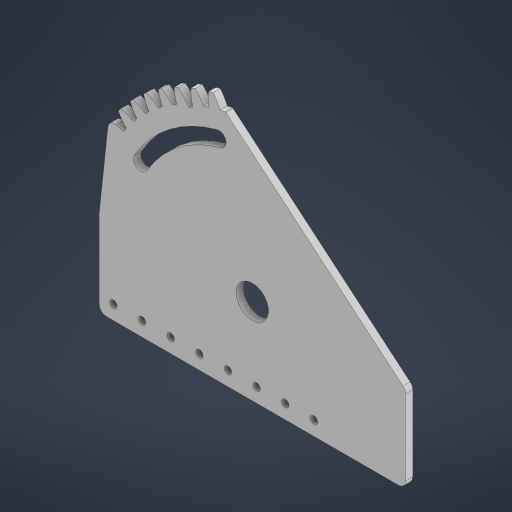
# Autodesk Inventor part: SHOT_0_001
Saved by Autodesk Inventor 2024.2 (Build 282272000, 272)
## iProperties
Created: 2024-08-07
Part Number: SHOT_0_001
Material: Generic
Document SubType Name: Modeling
Designer: Bryan
Density: 1 g/cm^3
Appearance: Default
Author: Bryan
Autodesk Inventor part; units mm, degrees
ref_plane "YZ Plane" through (0, 0, 0) normal (1, 0, 0) x (0, 1, 0)
ref_plane "XZ Plane" through (0, 0, 0) normal (0, 1, 0) x (-1, 0, 0)
ref_plane "XY Plane" through (0, 0, 0) normal (0, 0, 1) x (1, 0, 0)
sketch "Sketch2" plane through (0, 0, 0) normal (0, 0, 1) x (1, 0, 0)
  circle A0 centre (0, 0) radius 142.24 construction
  circle A1 centre (0, 0) radius 135.89
  circle A2 centre (0, 0) radius 147.32
  line L0 (0, 142.24) -> (0, 0) construction
  line L1 (0, 0) -> (-45.7151, 125.6011) construction
  line L2 (-45.7151, 125.6011) -> (0, 142.24) construction
  arc A3 (1.9921, 133.647) -> (-45.7151, 125.6011) centre (0, 0) ccw construction
  arc A4 (-45.7151, 125.6011) -> (-57.9663, 120.4384) centre (0, 0) ccw
  line L3 (-57.9663, 120.4384) -> (-2.146, 147.3044) construction
  spline S0 degree 2 poles (-2.146, 147.3044) (0.5723, 142.4261) (1.9921, 133.647) knots 0 0 0 1 1 1
  line L4 (0, 0) -> (3.8112, 135.8365) construction
  spline S1 degree 2 poles (10.4021, 146.9523) (7.4145, 142.2341) (5.5047, 133.5485) knots 0 0 0 1 1 1
  spline S2 degree 2 poles (-18.6254, 146.1379) (-15.3779, 141.5946) (-12.9842, 133.0297) knots 0 0 0 1 1 1
  spline S3 degree 2 poles (-6.1168, 147.193) (-8.5573, 142.1699) (-9.4826, 133.3251) knots 0 0 0 1 1 1
  spline S4 degree 2 poles (-34.8705, 143.1336) (-31.1348, 138.9825) (-27.7971, 130.7395) knots 0 0 0 1 1 1
  spline S5 degree 2 poles (-22.5587, 145.5826) (-24.4215, 140.3178) (-24.3506, 131.4251) knots 0 0 0 1 1 1
  spline S6 degree 2 poles (-50.6772, 138.3293) (-46.5001, 134.6226) (-42.2605, 126.8051) knots 0 0 0 1 1 1
  spline S7 degree 2 poles (-38.7169, 142.1414) (-39.9785, 136.7012) (-38.9125, 127.8723) knots 0 0 0 1 1 1
  spline S8 degree 2 poles (-65.8465, 131.7855) (-61.2807, 128.5698) (-56.1925, 121.2761) knots 0 0 0 1 1 1
  spline S9 degree 2 poles (-54.3883, 136.9127) (-55.0328, 131.3655) (-52.9849, 122.7114) knots 0 0 0 1 1 1
  spline S10 degree 2 poles (-80.1878, 123.5844) (-75.2906, 120.9001) (-69.4178, 114.222) knots 0 0 0 1 1 1
  spline S11 degree 2 poles (-69.3756, 129.9623) (-69.3951, 124.3778) (-66.3911, 116.0074) knots 0 0 0 1 1 1
  spline S12 degree 2 poles (-93.5206, 113.8292) (-88.3537, 111.71) (-81.7701, 105.7315) knots 0 0 0 1 1 1
  spline S13 degree 2 poles (-83.4906, 121.3775) (-82.8846, 115.8259) (-78.9624, 107.8445) knots 0 0 0 1 1 1
  spline S14 degree 2 poles (-105.6774, 102.6424) (-100.3057, 101.1151) (-93.0941, 95.9113) knots 0 0 0 1 1 1
  spline S15 degree 2 poles (-96.5556, 111.2664) (-95.3319, 105.8175) (-90.5406, 98.3255) knots 0 0 0 1 1 1
  spline S16 degree 2 poles (-116.5052, 90.1649) (-110.9963, 89.2486) (-103.2474, 84.885) knots 0 0 0 1 1 1
  spline S17 degree 2 poles (-108.4063, 99.7559) (-106.5802, 94.4784) (-100.9803, 87.5699) knots 0 0 0 1 1 1
  spline S18 degree 2 poles (-125.8679, 76.5535) (-120.2911, 76.2598) (-112.1023, 72.7912) knots 0 0 0 1 1 1
  spline S19 degree 2 poles (-118.8938, 86.991) (-116.4883, 81.9511) (-110.15, 75.713) knots 0 0 0 1 1 1
  spline S20 degree 2 poles (-133.6478, 61.9795) (-128.0731, 62.312) (-119.5475, 59.7821) knots 0 0 0 1 1 1
  spline S21 degree 2 poles (-127.8862, 73.1322) (-124.9315, 68.3933) (-117.9346, 62.9041) knots 0 0 0 1 1 1
  spline S22 degree 2 poles (-139.7469, 46.6259) (-134.2446, 47.5805) (-125.4893, 46.0211) knots 0 0 0 1 1 1
  spline S23 degree 2 poles (-135.2702, 58.3536) (-131.8035, 53.9753) (-124.2361, 49.3041) knots 0 0 0 1 1 1
  spline S24 degree 2 poles (-144.0887, 30.6861) (-138.7278, 32.2507) (-129.8529, 31.6814) knots 0 0 0 1 1 1
  spline S25 degree 2 poles (-140.9532, 42.8412) (-137.0181, 38.8786) (-128.9752, 35.084) knots 0 0 0 1 1 1
  spline S26 degree 2 poles (-146.6184, 14.3603) (-141.4664, 16.5154) (-132.5836, 16.9433) knots 0 0 0 1 1 1
  spline S27 degree 2 poles (-144.8636, 26.7901) (-140.5096, 23.293) (-132.0924, 20.4228) knots 0 0 0 1 1 1
  spline S28 degree 2 poles (-147.3044, -2.146) (-142.4261, 0.5723) (-133.647, 1.9921) knots 0 0 0 1 1 1
  spline S29 degree 2 poles (-146.9523, 10.4021) (-142.2341, 7.4145) (-133.5485, 5.5047) knots 0 0 0 1 1 1
  spline S30 degree 2 poles (-146.1379, -18.6254) (-141.5946, -15.3779) (-133.0297, -12.9842) knots 0 0 0 1 1 1
  spline S31 degree 2 poles (-147.193, -6.1168) (-142.1699, -8.5573) (-133.3251, -9.4826) knots 0 0 0 1 1 1
  spline S32 degree 2 poles (-143.1336, -34.8705) (-138.9825, -31.1348) (-130.7395, -27.7971) knots 0 0 0 1 1 1
  spline S33 degree 2 poles (-145.5826, -22.5587) (-140.3178, -24.4215) (-131.4251, -24.3506) knots 0 0 0 1 1 1
  spline S34 degree 2 poles (-138.3293, -50.6772) (-134.6226, -46.5001) (-126.8051, -42.2605) knots 0 0 0 1 1 1
  spline S35 degree 2 poles (-142.1414, -38.7169) (-136.7012, -39.9785) (-127.8723, -38.9125) knots 0 0 0 1 1 1
  spline S36 degree 2 poles (-131.7855, -65.8465) (-128.5698, -61.2807) (-121.2761, -56.1925) knots 0 0 0 1 1 1
  spline S37 degree 2 poles (-136.9127, -54.3883) (-131.3655, -55.0328) (-122.7114, -52.9849) knots 0 0 0 1 1 1
  spline S38 degree 2 poles (-123.5844, -80.1878) (-120.9001, -75.2906) (-114.222, -69.4178) knots 0 0 0 1 1 1
  spline S39 degree 2 poles (-129.9623, -69.3756) (-124.3778, -69.3951) (-116.0074, -66.3911) knots 0 0 0 1 1 1
  spline S40 degree 2 poles (-113.8292, -93.5206) (-111.71, -88.3537) (-105.7315, -81.7701) knots 0 0 0 1 1 1
  spline S41 degree 2 poles (-121.3775, -83.4906) (-115.8259, -82.8846) (-107.8445, -78.9624) knots 0 0 0 1 1 1
  spline S42 degree 2 poles (-102.6424, -105.6774) (-101.1151, -100.3057) (-95.9113, -93.0941) knots 0 0 0 1 1 1
  spline S43 degree 2 poles (-111.2664, -96.5556) (-105.8175, -95.3319) (-98.3255, -90.5406) knots 0 0 0 1 1 1
  spline S44 degree 2 poles (-90.1649, -116.5052) (-89.2486, -110.9963) (-84.885, -103.2474) knots 0 0 0 1 1 1
  spline S45 degree 2 poles (-99.7559, -108.4063) (-94.4784, -106.5802) (-87.5699, -100.9803) knots 0 0 0 1 1 1
  spline S46 degree 2 poles (-76.5535, -125.8679) (-76.2598, -120.2911) (-72.7912, -112.1023) knots 0 0 0 1 1 1
  spline S47 degree 2 poles (-86.991, -118.8938) (-81.9511, -116.4883) (-75.713, -110.15) knots 0 0 0 1 1 1
  spline S48 degree 2 poles (-61.9795, -133.6478) (-62.312, -128.0731) (-59.7821, -119.5475) knots 0 0 0 1 1 1
  spline S49 degree 2 poles (-73.1322, -127.8862) (-68.3933, -124.9315) (-62.9041, -117.9346) knots 0 0 0 1 1 1
  spline S50 degree 2 poles (-46.6259, -139.7469) (-47.5805, -134.2446) (-46.0211, -125.4893) knots 0 0 0 1 1 1
  spline S51 degree 2 poles (-58.3536, -135.2702) (-53.9753, -131.8035) (-49.3041, -124.2361) knots 0 0 0 1 1 1
  spline S52 degree 2 poles (-30.6861, -144.0887) (-32.2507, -138.7278) (-31.6814, -129.8529) knots 0 0 0 1 1 1
  spline S53 degree 2 poles (-42.8412, -140.9532) (-38.8786, -137.0181) (-35.084, -128.9752) knots 0 0 0 1 1 1
  spline S54 degree 2 poles (-14.3603, -146.6184) (-16.5154, -141.4664) (-16.9433, -132.5836) knots 0 0 0 1 1 1
  spline S55 degree 2 poles (-26.7901, -144.8636) (-23.293, -140.5096) (-20.4228, -132.0924) knots 0 0 0 1 1 1
  spline S56 degree 2 poles (2.146, -147.3044) (-0.5723, -142.4261) (-1.9921, -133.647) knots 0 0 0 1 1 1
  spline S57 degree 2 poles (-10.4021, -146.9523) (-7.4145, -142.2341) (-5.5047, -133.5485) knots 0 0 0 1 1 1
  spline S58 degree 2 poles (18.6254, -146.1379) (15.3779, -141.5946) (12.9842, -133.0297) knots 0 0 0 1 1 1
  spline S59 degree 2 poles (6.1168, -147.193) (8.5573, -142.1699) (9.4826, -133.3251) knots 0 0 0 1 1 1
  spline S60 degree 2 poles (34.8705, -143.1336) (31.1348, -138.9825) (27.7971, -130.7395) knots 0 0 0 1 1 1
  spline S61 degree 2 poles (22.5587, -145.5826) (24.4215, -140.3178) (24.3506, -131.4251) knots 0 0 0 1 1 1
  spline S62 degree 2 poles (50.6772, -138.3293) (46.5001, -134.6226) (42.2605, -126.8051) knots 0 0 0 1 1 1
  spline S63 degree 2 poles (38.7169, -142.1414) (39.9785, -136.7012) (38.9125, -127.8723) knots 0 0 0 1 1 1
  spline S64 degree 2 poles (65.8465, -131.7855) (61.2807, -128.5698) (56.1925, -121.2761) knots 0 0 0 1 1 1
  spline S65 degree 2 poles (54.3883, -136.9127) (55.0328, -131.3655) (52.9849, -122.7114) knots 0 0 0 1 1 1
  spline S66 degree 2 poles (80.1878, -123.5844) (75.2906, -120.9001) (69.4178, -114.222) knots 0 0 0 1 1 1
  spline S67 degree 2 poles (69.3756, -129.9623) (69.3951, -124.3778) (66.3911, -116.0074) knots 0 0 0 1 1 1
  spline S68 degree 2 poles (93.5206, -113.8292) (88.3537, -111.71) (81.7701, -105.7315) knots 0 0 0 1 1 1
  spline S69 degree 2 poles (83.4906, -121.3775) (82.8846, -115.8259) (78.9624, -107.8445) knots 0 0 0 1 1 1
  spline S70 degree 2 poles (105.6774, -102.6424) (100.3057, -101.1151) (93.0941, -95.9113) knots 0 0 0 1 1 1
  spline S71 degree 2 poles (96.5556, -111.2664) (95.3319, -105.8175) (90.5406, -98.3255) knots 0 0 0 1 1 1
  spline S72 degree 2 poles (116.5052, -90.1649) (110.9963, -89.2486) (103.2474, -84.885) knots 0 0 0 1 1 1
  spline S73 degree 2 poles (108.4063, -99.7559) (106.5802, -94.4784) (100.9803, -87.5699) knots 0 0 0 1 1 1
  spline S74 degree 2 poles (125.8679, -76.5535) (120.2911, -76.2598) (112.1023, -72.7912) knots 0 0 0 1 1 1
  spline S75 degree 2 poles (118.8938, -86.991) (116.4883, -81.9511) (110.15, -75.713) knots 0 0 0 1 1 1
  spline S76 degree 2 poles (133.6478, -61.9795) (128.0731, -62.312) (119.5475, -59.7821) knots 0 0 0 1 1 1
  spline S77 degree 2 poles (127.8862, -73.1322) (124.9315, -68.3933) (117.9346, -62.9041) knots 0 0 0 1 1 1
  spline S78 degree 2 poles (139.7469, -46.6259) (134.2446, -47.5805) (125.4893, -46.0211) knots 0 0 0 1 1 1
  spline S79 degree 2 poles (135.2702, -58.3536) (131.8035, -53.9753) (124.2361, -49.3041) knots 0 0 0 1 1 1
  spline S80 degree 2 poles (144.0887, -30.6861) (138.7278, -32.2507) (129.8529, -31.6814) knots 0 0 0 1 1 1
  spline S81 degree 2 poles (140.9532, -42.8412) (137.0181, -38.8786) (128.9752, -35.084) knots 0 0 0 1 1 1
  spline S82 degree 2 poles (146.6184, -14.3603) (141.4664, -16.5154) (132.5836, -16.9433) knots 0 0 0 1 1 1
  spline S83 degree 2 poles (144.8636, -26.7901) (140.5096, -23.293) (132.0924, -20.4228) knots 0 0 0 1 1 1
  spline S84 degree 2 poles (147.3044, 2.146) (142.4261, -0.5723) (133.647, -1.9921) knots 0 0 0 1 1 1
  spline S85 degree 2 poles (146.9523, -10.4021) (142.2341, -7.4145) (133.5485, -5.5047) knots 0 0 0 1 1 1
  spline S86 degree 2 poles (146.1379, 18.6254) (141.5946, 15.3779) (133.0297, 12.9842) knots 0 0 0 1 1 1
  spline S87 degree 2 poles (147.193, 6.1168) (142.1699, 8.5573) (133.3251, 9.4826) knots 0 0 0 1 1 1
  spline S88 degree 2 poles (143.1336, 34.8705) (138.9825, 31.1348) (130.7395, 27.7971) knots 0 0 0 1 1 1
  spline S89 degree 2 poles (145.5826, 22.5587) (140.3178, 24.4215) (131.4251, 24.3506) knots 0 0 0 1 1 1
  spline S90 degree 2 poles (138.3293, 50.6772) (134.6226, 46.5001) (126.8051, 42.2605) knots 0 0 0 1 1 1
  spline S91 degree 2 poles (142.1414, 38.7169) (136.7012, 39.9785) (127.8723, 38.9125) knots 0 0 0 1 1 1
  spline S92 degree 2 poles (131.7855, 65.8465) (128.5698, 61.2807) (121.2761, 56.1925) knots 0 0 0 1 1 1
  spline S93 degree 2 poles (136.9127, 54.3883) (131.3655, 55.0328) (122.7114, 52.9849) knots 0 0 0 1 1 1
  spline S94 degree 2 poles (123.5844, 80.1878) (120.9001, 75.2906) (114.222, 69.4178) knots 0 0 0 1 1 1
  spline S95 degree 2 poles (129.9623, 69.3756) (124.3778, 69.3951) (116.0074, 66.3911) knots 0 0 0 1 1 1
  spline S96 degree 2 poles (113.8292, 93.5206) (111.71, 88.3537) (105.7315, 81.7701) knots 0 0 0 1 1 1
  spline S97 degree 2 poles (121.3775, 83.4906) (115.8259, 82.8846) (107.8445, 78.9624) knots 0 0 0 1 1 1
  spline S98 degree 2 poles (102.6424, 105.6774) (101.1151, 100.3057) (95.9113, 93.0941) knots 0 0 0 1 1 1
  spline S99 degree 2 poles (111.2664, 96.5556) (105.8175, 95.3319) (98.3255, 90.5406) knots 0 0 0 1 1 1
  spline S100 degree 2 poles (90.1649, 116.5052) (89.2486, 110.9963) (84.885, 103.2474) knots 0 0 0 1 1 1
  spline S101 degree 2 poles (99.7559, 108.4063) (94.4784, 106.5802) (87.5699, 100.9803) knots 0 0 0 1 1 1
  spline S102 degree 2 poles (76.5535, 125.8679) (76.2598, 120.2911) (72.7912, 112.1023) knots 0 0 0 1 1 1
  spline S103 degree 2 poles (86.991, 118.8938) (81.9511, 116.4883) (75.713, 110.15) knots 0 0 0 1 1 1
  spline S104 degree 2 poles (61.9795, 133.6478) (62.312, 128.0731) (59.7821, 119.5475) knots 0 0 0 1 1 1
  spline S105 degree 2 poles (73.1322, 127.8862) (68.3933, 124.9315) (62.9041, 117.9346) knots 0 0 0 1 1 1
  spline S106 degree 2 poles (46.6259, 139.7469) (47.5805, 134.2446) (46.0211, 125.4893) knots 0 0 0 1 1 1
  spline S107 degree 2 poles (58.3536, 135.2702) (53.9753, 131.8035) (49.3041, 124.2361) knots 0 0 0 1 1 1
  spline S108 degree 2 poles (30.6861, 144.0887) (32.2507, 138.7278) (31.6814, 129.8529) knots 0 0 0 1 1 1
  spline S109 degree 2 poles (42.8412, 140.9532) (38.8786, 137.0181) (35.084, 128.9752) knots 0 0 0 1 1 1
  spline S110 degree 2 poles (14.3603, 146.6184) (16.5154, 141.4664) (16.9433, 132.5836) knots 0 0 0 1 1 1
  spline S111 degree 2 poles (26.7901, 144.8636) (23.293, 140.5096) (20.4228, 132.0924) knots 0 0 0 1 1 1
  circle A5 centre (0, 0) radius 6.35
  point P0 (7.9755, 142.0162)
  point P1 (-15.9258, 141.3456)
  point P2 (-7.9755, 142.0162)
  point P3 (-31.6514, 138.6737)
  point P4 (-23.8261, 140.2303)
  point P5 (-46.9789, 134.258)
  point P6 (-39.3771, 136.6809)
  point P7 (-61.7156, 128.1538)
  point P8 (-54.4329, 131.4126)
  point P9 (-75.6762, 120.4381)
  point P10 (-68.8042, 124.4918)
  point P11 (-88.6852, 111.2077)
  point P12 (-82.3102, 116.0054)
  point P13 (-100.5789, 100.5789)
  point P14 (-94.7811, 106.0601)
  point P15 (-111.2077, 88.6852)
  point P16 (-106.0601, 94.7811)
  point P17 (-120.4381, 75.6762)
  point P18 (-116.0054, 82.3102)
  point P19 (-128.1538, 61.7156)
  point P20 (-124.4918, 68.8042)
  point P21 (-134.258, 46.9789)
  point P22 (-131.4126, 54.4329)
  point P23 (-138.6737, 31.6514)
  point P24 (-136.6809, 39.3771)
  point P25 (-141.3456, 15.9258)
  point P26 (-140.2303, 23.8261)
  point P27 (-142.24, 0)
  point P28 (-142.0162, 7.9755)
  point P29 (-141.3456, -15.9258)
  point P30 (-142.0162, -7.9755)
  point P31 (-138.6737, -31.6514)
  point P32 (-140.2303, -23.8261)
  point P33 (-134.258, -46.9789)
  point P34 (-136.6809, -39.3771)
  point P35 (-128.1538, -61.7156)
  point P36 (-131.4126, -54.4329)
  point P37 (-120.4381, -75.6762)
  point P38 (-124.4918, -68.8042)
  point P39 (-111.2077, -88.6852)
  point P40 (-116.0054, -82.3102)
  point P41 (-100.5789, -100.5789)
  point P42 (-106.0601, -94.7811)
  point P43 (-88.6852, -111.2077)
  point P44 (-94.7811, -106.0601)
  point P45 (-75.6762, -120.4381)
  point P46 (-82.3102, -116.0054)
  point P47 (-61.7156, -128.1538)
  point P48 (-68.8042, -124.4918)
  point P49 (-46.9789, -134.258)
  point P50 (-54.4329, -131.4126)
  point P51 (-31.6514, -138.6737)
  point P52 (-39.3771, -136.6809)
  point P53 (-15.9258, -141.3456)
  point P54 (-23.8261, -140.2303)
  point P55 (0, -142.24)
  point P56 (-7.9755, -142.0162)
  point P57 (15.9258, -141.3456)
  point P58 (7.9755, -142.0162)
  point P59 (31.6514, -138.6737)
  point P60 (23.8261, -140.2303)
  point P61 (46.9789, -134.258)
  point P62 (39.3771, -136.6809)
  point P63 (61.7156, -128.1538)
  point P64 (54.4329, -131.4126)
  point P65 (75.6762, -120.4381)
  point P66 (68.8042, -124.4918)
  point P67 (88.6852, -111.2077)
  point P68 (82.3102, -116.0054)
  point P69 (100.5789, -100.5789)
  point P70 (94.7811, -106.0601)
  point P71 (111.2077, -88.6852)
  point P72 (106.0601, -94.7811)
  point P73 (120.4381, -75.6762)
  point P74 (116.0054, -82.3102)
  point P75 (128.1538, -61.7156)
  point P76 (124.4918, -68.8042)
  point P77 (134.258, -46.9789)
  point P78 (131.4126, -54.4329)
  point P79 (138.6737, -31.6514)
  point P80 (136.6809, -39.3771)
  point P81 (141.3456, -15.9258)
  point P82 (140.2303, -23.8261)
  point P83 (142.24, 0)
  point P84 (142.0162, -7.9755)
  point P85 (141.3456, 15.9258)
  point P86 (142.0162, 7.9755)
  point P87 (138.6737, 31.6514)
  point P88 (140.2303, 23.8261)
  point P89 (134.258, 46.9789)
  point P90 (136.6809, 39.3771)
  point P91 (128.1538, 61.7156)
  point P92 (131.4126, 54.4329)
  point P93 (120.4381, 75.6762)
  point P94 (124.4918, 68.8042)
  point P95 (111.2077, 88.6852)
  point P96 (116.0054, 82.3102)
  point P97 (100.5789, 100.5789)
  point P98 (106.0601, 94.7811)
  point P99 (88.6852, 111.2077)
  point P100 (94.7811, 106.0601)
  point P101 (75.6762, 120.4381)
  point P102 (82.3102, 116.0054)
  point P103 (61.7156, 128.1538)
  point P104 (68.8042, 124.4918)
  point P105 (46.9789, 134.258)
  point P106 (54.4329, 131.4126)
  point P107 (31.6514, 138.6737)
  point P108 (39.3771, 136.6809)
  point P109 (15.9258, 141.3456)
  point P110 (23.8261, 140.2303)
  point P111 (-52.9849, 122.7114)
  point P112 (-56.1925, 121.2761)
  point P113 (-65.8465, 131.7855)
  point P114 (-67.1264, 118.153)
  point P115 (-70.94, 115.9034)
  point P116 (-80.1878, 123.5844)
  point P117 (-79.9333, 109.8943)
  point P118 (-83.471, 107.2319)
  point P119 (-93.5206, 113.8292)
  point P120 (-96.5556, 111.2664)
  point P121 (-91.7349, 100.2537)
  point P122 (-94.9523, 97.2119)
  point P123 (-108.4063, 99.7559)
  point P124 (-102.383, 89.3522)
  point P125 (-105.2396, 85.9693)
  point P126 (-116.5052, 90.1649)
  point P127 (-118.8938, 86.991)
  point P128 (-111.7435, 77.3272)
  point P129 (-114.2034, 73.6457)
  point P130 (-125.8679, 76.5535)
  point P131 (-127.8862, 73.1322)
  point P132 (-119.6987, 64.3296)
  point P133 (-121.731, 60.3959)
  point P134 (-133.6478, 61.9795)
  point P135 (-135.2702, 58.3536)
  point P136 (-126.1487, 50.5231)
  point P137 (-127.7277, 46.3866)
  point P138 (-139.7469, 46.6259)
  point P139 (-140.9532, 42.8412)
  point P140 (-131.0123, 36.0813)
  point P141 (-132.1183, 31.794)
  point P142 (-144.0887, 30.6861)
  point P143 (-144.8636, 26.7901)
  point P144 (-134.2284, 21.1857)
  point P145 (-134.8473, 16.8015)
  point P146 (-146.6184, 14.3603)
  point P147 (-135.7564, 6.0237)
  point P148 (123.1174, 57.5169)
  point P149 (131.7855, 65.8465)
  point P150 (129.9623, 69.3756)
  point P151 (118.153, 67.1264)
  point P152 (115.9034, 70.94)
  point P153 (123.5844, 80.1878)
  point P154 (121.3775, 83.4906)
  point P155 (109.8943, 79.9333)
  point P156 (107.2319, 83.471)
  point P157 (113.8292, 93.5206)
  point P158 (111.2664, 96.5556)
  point P159 (100.2537, 91.7349)
  point P160 (97.2119, 94.9523)
  point P161 (102.6424, 105.6774)
  point P162 (99.7559, 108.4063)
  point P163 (89.3522, 102.383)
  point P164 (85.9693, 105.2396)
  point P165 (90.1649, 116.5052)
  point P166 (86.991, 118.8938)
  point P167 (77.3272, 111.7435)
  point P168 (73.6457, 114.2034)
  point P169 (76.5535, 125.8679)
  point P170 (73.1322, 127.8862)
  point P171 (64.3296, 119.6987)
  point P172 (60.3959, 121.731)
  point P173 (61.9795, 133.6478)
  point P174 (58.3536, 135.2702)
  point P175 (50.5231, 126.1487)
  point P176 (46.3866, 127.7277)
  point P177 (46.6259, 139.7469)
  point P178 (42.8412, 140.9532)
  point P179 (36.0813, 131.0123)
  point P180 (31.794, 132.1183)
  point P181 (30.6861, 144.0887)
  point P182 (26.7901, 144.8636)
  point P183 (21.1857, 134.2284)
  point P184 (16.8015, 134.8473)
  point P185 (14.3603, 146.6184)
  point P186 (6.0237, 135.7564)
  point P187 (1.5977, 135.8806)
  point P188 (-6.1168, 147.193)
  point P189 (-9.2141, 135.5773)
  point P190 (-13.6261, 135.2051)
  point P191 (-18.6254, 146.1379)
  point P192 (-24.336, 133.6931)
  point P193 (-28.6786, 132.8293)
  point P194 (-34.8705, 143.1336)
  point P195 (-39.1519, 130.1277)
  point P196 (-43.3704, 128.7831)
  point P197 (-50.6772, 138.3293)
  point P198 (-54.3883, 136.9127)
  dimension "d0" = 284.48
  dimension "d1" = 271.78
  dimension "d2" = 294.64
  dimension "d3" = 20
  dimension "d4" = 48.6489
  dimension "d5" = 48.6489
  dimension "d6" = 61.949
  dimension "d7" = 13.3001
  dimension "d8" = 1.607
  dimension "d11" = 360
  dimension "d13" = 12.7
  constraints: 10 end point, 4 coincident, 4 point on circle, 3 centre point, 3 symmetric about line, 1 perpendicular, 1 tangent, 1 vertical, 1 vertical alignment, 795 other
  measures "d3" angle of L0 L1
  measures "d4" distance of L1.end L0.start
  measures "d6" distance of L3.start L3.end
  measures "d8" angle of L4 L0
  measures "d13" diameter of A5
extrude "Extrusion1" add sketch "Sketch2" along normal blind 6.35 contours A1 S8 A4 S9 | A1 S95 A2 S92 | A1 S97 A2 S94 | A1 S99 A2 S96 | A1 S101 A2 S98 | A1 S103 A2 S100 | A1 S105 A2 S102 | A1 S107 A2 S104 | A1 S109 A2 S106 | A1 S111 A2 S108 | A1 S1 A2 S110 | A1 S3 A2 S0 | A1 S5 A2 S2 | A1 S7 A2 S4 | A1 S9 A2 S6 | A1 S11 A2 S8 | A1 S13 A2 S10 | A1 S15 A2 S12 | A1 S17 A2 S14 | A1 S19 A2 S16 | A1 S21 A2 S18 | A1 S23 A2 S20 | A1 S25 A2 S22 | A1 S27 A2 S24 | A1 S29 A2 S26 picked at (-28.6478, 87.0122)
sketch "Sketch3" plane through (0, 0, 6.35) normal (0, 0, 1) x (1, 0, 0)
  circle A0 centre (0, 0) radius 6.35 projected
  line L0 (0, 0) -> (-127.5829, 73.66)
  line L1 (0, 0) -> (-25.5818, 145.0819)
  line L2 (0, 0) -> (-135.89, 0) construction
  arc A1 (-135.7564, 6.0237) -> (123.1174, 57.5169) centre (0, 0) ccw projected
  line L3 (-135.89, 0) -> (-135.89, -76.2)
  line L4 (135.89, 0) -> (135.89, -76.2)
  line L5 (-135.89, -50.8) -> (135.89, -50.8)
  line L6 (-135.89, -76.2) -> (135.89, -76.2)
  arc A2 (-52.9849, 122.7114) -> (-56.1925, 121.2761) centre (0, 0) ccw projected
  arc A3 (-65.8465, 131.7855) -> (-69.3756, 129.9623) centre (0, 0) ccw projected
  arc A4 (-67.1264, 118.153) -> (-70.94, 115.9034) centre (0, 0) ccw projected
  arc A5 (-80.1878, 123.5844) -> (-83.4906, 121.3775) centre (0, 0) ccw projected
  arc A6 (-79.9333, 109.8943) -> (-83.471, 107.2319) centre (0, 0) ccw projected
  arc A7 (-93.5206, 113.8292) -> (-96.5556, 111.2664) centre (0, 0) ccw projected
  arc A8 (-91.7349, 100.2537) -> (-94.9523, 97.2119) centre (0, 0) ccw projected
  arc A9 (-105.6774, 102.6424) -> (-108.4063, 99.7559) centre (0, 0) ccw projected
  arc A10 (-102.383, 89.3522) -> (-105.2396, 85.9693) centre (0, 0) ccw projected
  arc A11 (-116.5052, 90.1649) -> (-118.8938, 86.991) centre (0, 0) ccw projected
  arc A12 (-111.7435, 77.3272) -> (-114.2034, 73.6457) centre (0, 0) ccw projected
  arc A13 (-125.8679, 76.5535) -> (-127.8862, 73.1322) centre (0, 0) ccw projected
  spline S0 degree 2 poles (-127.8862, 73.1322) (-125.3186, 69.0142) (-119.6987, 64.3296) knots 0 0 0 1 1 1 projected
  arc A14 (-119.6987, 64.3296) -> (-121.731, 60.3959) centre (0, 0) ccw projected
  spline S1 degree 2 poles (-121.731, 60.3959) (-128.8035, 62.2684) (-133.6478, 61.9795) knots 0 0 0 1 1 1 projected
  arc A15 (-133.6478, 61.9795) -> (-135.2702, 58.3536) centre (0, 0) ccw projected
  spline S2 degree 2 poles (-135.2702, 58.3536) (-132.2578, 54.549) (-126.1487, 50.5231) knots 0 0 0 1 1 1 projected
  arc A16 (-126.1487, 50.5231) -> (-127.7277, 46.3866) centre (0, 0) ccw projected
  spline S3 degree 2 poles (-127.7277, 46.3866) (-134.9655, 47.4555) (-139.7469, 46.6259) knots 0 0 0 1 1 1 projected
  arc A17 (-139.7469, 46.6259) -> (-140.9532, 42.8412) centre (0, 0) ccw projected
  spline S4 degree 2 poles (-140.9532, 42.8412) (-137.5337, 39.3978) (-131.0123, 36.0813) knots 0 0 0 1 1 1 projected
  arc A18 (-131.0123, 36.0813) -> (-132.1183, 31.794) centre (0, 0) ccw projected
  spline S5 degree 2 poles (-132.1183, 31.794) (-139.4302, 32.0457) (-144.0887, 30.6861) knots 0 0 0 1 1 1 projected
  arc A19 (-144.0887, 30.6861) -> (-144.8636, 26.7901) centre (0, 0) ccw projected
  spline S6 degree 2 poles (-144.8636, 26.7901) (-141.0801, 23.7512) (-134.2284, 21.1857) knots 0 0 0 1 1 1 projected
  arc A20 (-134.2284, 21.1857) -> (-134.8473, 16.8015) centre (0, 0) ccw projected
  spline S7 degree 2 poles (-134.8473, 16.8015) (-142.1415, 16.233) (-146.6184, 14.3603) knots 0 0 0 1 1 1 projected
  arc A21 (-146.6184, 14.3603) -> (-146.9523, 10.4021) centre (0, 0) ccw projected
  spline S8 degree 2 poles (-146.9523, 10.4021) (-142.8523, 7.8059) (-135.7564, 6.0237) knots 0 0 0 1 1 1 projected
  arc A22 (-135.7564, 6.0237) -> (123.1174, 57.5169) centre (0, 0) ccw projected
  spline S9 degree 2 poles (123.1174, 57.5169) (128.9911, 61.8789) (131.7855, 65.8465) knots 0 0 0 1 1 1 projected
  arc A23 (131.7855, 65.8465) -> (129.9623, 69.3756) centre (0, 0) ccw projected
  spline S10 degree 2 poles (129.9623, 69.3756) (125.1095, 69.3925) (118.153, 67.1264) knots 0 0 0 1 1 1 projected
  arc A24 (118.153, 67.1264) -> (115.9034, 70.94) centre (0, 0) ccw projected
  spline S11 degree 2 poles (115.9034, 70.94) (121.2518, 75.9323) (123.5844, 80.1878) knots 0 0 0 1 1 1 projected
  arc A25 (123.5844, 80.1878) -> (121.3775, 83.4906) centre (0, 0) ccw projected
  spline S12 degree 2 poles (121.3775, 83.4906) (116.5533, 82.964) (109.8943, 79.9333) knots 0 0 0 1 1 1 projected
  arc A26 (109.8943, 79.9333) -> (107.2319, 83.471) centre (0, 0) ccw projected
  spline S13 degree 2 poles (107.2319, 83.471) (111.9877, 89.0307) (113.8292, 93.5206) knots 0 0 0 1 1 1 projected
  arc A27 (113.8292, 93.5206) -> (111.2664, 96.5556) centre (0, 0) ccw projected
  spline S14 degree 2 poles (111.2664, 96.5556) (106.5314, 95.4922) (100.2537, 91.7349) knots 0 0 0 1 1 1 projected
  arc A28 (100.2537, 91.7349) -> (97.2119, 94.9523) centre (0, 0) ccw projected
  spline S15 degree 2 poles (97.2119, 94.9523) (101.3152, 101.0096) (102.6424, 105.6774) knots 0 0 0 1 1 1 projected
  arc A29 (102.6424, 105.6774) -> (99.7559, 108.4063) centre (0, 0) ccw projected
  spline S16 degree 2 poles (99.7559, 108.4063) (95.1699, 106.8195) (89.3522, 102.383) knots 0 0 0 1 1 1 projected
  arc A30 (89.3522, 102.383) -> (85.9693, 105.2396) centre (0, 0) ccw projected
  spline S17 degree 2 poles (85.9693, 105.2396) (89.3687, 111.7181) (90.1649, 116.5052) knots 0 0 0 1 1 1 projected
  arc A31 (90.1649, 116.5052) -> (86.991, 118.8938) centre (0, 0) ccw projected
  spline S18 degree 2 poles (86.991, 118.8938) (82.6115, 116.8035) (77.3272, 111.7435) knots 0 0 0 1 1 1 projected
  arc A32 (77.3272, 111.7435) -> (73.6457, 114.2034) centre (0, 0) ccw projected
  spline S19 degree 2 poles (73.6457, 114.2034) (76.2983, 121.0218) (76.5535, 125.8679) knots 0 0 0 1 1 1 projected
  arc A33 (76.5535, 125.8679) -> (73.1322, 127.8862) centre (0, 0) ccw projected
  spline S20 degree 2 poles (73.1322, 127.8862) (69.0142, 125.3186) (64.3296, 119.6987) knots 0 0 0 1 1 1 projected
  arc A34 (64.3296, 119.6987) -> (60.3959, 121.731) centre (0, 0) ccw projected
  spline S21 degree 2 poles (60.3959, 121.731) (62.2684, 128.8035) (61.9795, 133.6478) knots 0 0 0 1 1 1 projected
  arc A35 (61.9795, 133.6478) -> (58.3536, 135.2702) centre (0, 0) ccw projected
  spline S22 degree 2 poles (58.3536, 135.2702) (54.549, 132.2578) (50.5231, 126.1487) knots 0 0 0 1 1 1 projected
  arc A36 (50.5231, 126.1487) -> (46.3866, 127.7277) centre (0, 0) ccw projected
  spline S23 degree 2 poles (46.3866, 127.7277) (47.4555, 134.9655) (46.6259, 139.7469) knots 0 0 0 1 1 1 projected
  arc A37 (46.6259, 139.7469) -> (42.8412, 140.9532) centre (0, 0) ccw projected
  spline S24 degree 2 poles (42.8412, 140.9532) (39.3978, 137.5337) (36.0813, 131.0123) knots 0 0 0 1 1 1 projected
  arc A38 (36.0813, 131.0123) -> (31.794, 132.1183) centre (0, 0) ccw projected
  spline S25 degree 2 poles (31.794, 132.1183) (32.0457, 139.4302) (30.6861, 144.0887) knots 0 0 0 1 1 1 projected
  arc A39 (30.6861, 144.0887) -> (26.7901, 144.8636) centre (0, 0) ccw projected
  spline S26 degree 2 poles (26.7901, 144.8636) (23.7512, 141.0801) (21.1857, 134.2284) knots 0 0 0 1 1 1 projected
  arc A40 (21.1857, 134.2284) -> (16.8015, 134.8473) centre (0, 0) ccw projected
  spline S27 degree 2 poles (16.8015, 134.8473) (16.233, 142.1415) (14.3603, 146.6184) knots 0 0 0 1 1 1 projected
  arc A41 (14.3603, 146.6184) -> (10.4021, 146.9523) centre (0, 0) ccw projected
  spline S28 degree 2 poles (10.4021, 146.9523) (7.8059, 142.8523) (6.0237, 135.7564) knots 0 0 0 1 1 1 projected
  arc A42 (6.0237, 135.7564) -> (1.5977, 135.8806) centre (0, 0) ccw projected
  spline S29 degree 2 poles (1.5977, 135.8806) (0.2161, 143.0652) (-2.146, 147.3044) knots 0 0 0 1 1 1 projected
  arc A43 (-2.146, 147.3044) -> (-6.1168, 147.193) centre (0, 0) ccw projected
  spline S30 degree 2 poles (-6.1168, 147.193) (-8.2375, 142.828) (-9.2141, 135.5773) knots 0 0 0 1 1 1 projected
  arc A44 (-9.2141, 135.5773) -> (-13.6261, 135.2051) centre (0, 0) ccw projected
  spline S31 degree 2 poles (-13.6261, 135.2051) (-15.8034, 142.1899) (-18.6254, 146.1379) knots 0 0 0 1 1 1 projected
  arc A45 (-18.6254, 146.1379) -> (-22.5587, 145.5826) centre (0, 0) ccw projected
  spline S32 degree 2 poles (-22.5587, 145.5826) (-24.1774, 141.0077) (-24.336, 133.6931) knots 0 0 0 1 1 1 projected
  arc A46 (-24.336, 133.6931) -> (-28.6786, 132.8293) centre (0, 0) ccw projected
  arc A47 (-34.8705, 143.1336) -> (-38.7169, 142.1414) centre (0, 0) ccw projected
  arc A48 (-39.1519, 130.1277) -> (-43.3704, 128.7831) centre (0, 0) ccw projected
  arc A49 (-50.6772, 138.3293) -> (-54.3883, 136.9127) centre (0, 0) ccw projected
  circle A50 centre (0, 0) radius 6.35 projected
  line L7 (-127.8862, 73.1322) -> (-135.89, 0)
  line L8 (-23.5364, 133.4817) -> (135.89, 0)
  arc A51 (-23.5364, 133.4817) -> (-24.336, 133.6931) centre (-24.1616, 132.735) ccw
  point P0 (112.5151, -76.2)
  point P1 (-112.5151, -76.2)
  point P2 (-24.1725, 137.089)
  point P3 (123.1174, 57.5169)
  point P4 (-132.4093, 31.8034)
  point P5 (-129.1227, 61.8341)
  point P6 (-131.8913, 36.5363)
  point P7 (-130.0544, 53.3209)
  point P8 (-130.7721, 46.7629)
  dimension "d16" = 147.32
  dimension "d17" = 30
  dimension "d18" = 80
  dimension "d20" = 25.4
  dimension "d21" = 50.8
  constraints: 18 end point, 5 point on circle, 4 point on line, 3 horizontal, 3 tangent, 2 vertical, 1 centre point, 1 equal length, 48 other
  measures "d16" distance of L0.start L0.end
  measures "d17" angle of L2 L0
  measures "d18" angle of L1 L2
  measures "d20" distance between parallel lines of L6 L5
  measures "d21" distance from line of L5 point (0, 0)
extrude "Extrusion2" cut sketch "Sketch3" against normal blind 6.35 contours A51 S32 L1 | L1 S32 A45 S31 A44 S30 A43 S29 A42 S28 A41 S27 A40 S26 A39 S25 A38 S24 A37 S23 A36 S22 A35 S21 A34 S20 A33 S19 A32 S18 A31 S17 A30 S16 A29 S15 A28 S14 A27 S13 A26 S12 A25 S11 A24 S10 A23 S9 A1 L8 | A1 L6 | A1 S8 A21 S7 A20 S6 A19 S5 L7
extrude "Extrusion3" add sketch "Sketch3" against normal blind 6.35 contours L4 L5 A1 | L5 L4 L6 A1 | L5 L3 A1 | A1 L6 L3 L5
extrude "Extrusion4" add sketch "Sketch3" against normal blind 6.35 contours S0 A14 S1 L7 | S2 A16 S3 L7 | L7 S4 A18 S5
extrude "Extrusion5" cut sketch "Sketch3" against normal blind 6.35 contours L7 S2 A15 S1 | L7 S4 A17 S3
sketch "Sketch4" plane through (0, 0, 0) normal (0, 0, -1) x (-1, 0, 0)
  circle A0 centre (0, 0) radius 14.2875
  dimension "d30" = 28.575
  constraints: 1 centre point, 1 coincident
  measures "d30" diameter of A0
extrude "Extrusion6" cut sketch "Sketch4" against normal blind 6.35
fillet "Fillet1" radius 6.35 5 edges at (135.89, -76.2, 3.175) (-135.89, -76.2, 3.175) (135.89, 0, 3.175) (-127.8862, 73.1322, 3.175) (-125.8679, 76.5535, 3.175)
fillet "Fillet2" radius 25.4 1 edges at (-135.89, 0, 3.175)
sketch "Sketch5" plane through (0, 0, 6.35) normal (0, 0, 1) x (1, 0, 0)
  arc A0 (-29.583, 110.4053) -> (-98.9867, 57.15) centre (0, 0) ccw construction
  arc A1 (-31.2265, 116.539) -> (-104.486, 60.325) centre (0, 0) ccw
  arc A2 (-27.9395, 104.2717) -> (-93.4874, 53.975) centre (0, 0) ccw
  arc A3 (-27.9395, 104.2717) -> (-31.2265, 116.539) centre (-29.583, 110.4053) ccw
  arc A4 (-104.486, 60.325) -> (-93.4874, 53.975) centre (-98.9867, 57.15) ccw
  line L0 (0, 0) -> (-98.9867, 57.15) construction
  line L1 (0, 0) -> (114.3, 0) construction
  line L2 (0, 0) -> (-29.583, 110.4053) construction
  dimension "d35" = 114.3
  dimension "d36" = 150
  dimension "d37" = 45
  dimension "d38" = 12.7
  constraints: 10 point on circle, 6 end point, 5 centre point, 4 tangent, 1 coincident, 1 equal length, 1 horizontal
  measures "d35" radius of A0
  measures "d36" angle of L1 L0
  measures "d37" angle of L2 L0
  measures "d38" diameter of A3
extrude "Extrusion7" cut sketch "Sketch5" against normal blind 6.35
sketch "Sketch6" plane through (0, 0, 6.35) normal (0, 0, 1) x (1, 0, 0)
  circle A0 centre (-123.19, -63.5) radius 3.2512
  line L0 (-129.54, -76.2) -> (129.54, -76.2) projected
  line L1 (-135.89, -1.3858) -> (-135.89, -69.85) projected
  circle A1 centre (-97.79, -63.5) radius 3.2512
  circle A2 centre (-72.39, -63.5) radius 3.2512
  circle A3 centre (-46.99, -63.5) radius 3.2512
  circle A4 centre (-21.59, -63.5) radius 3.2512
  circle A5 centre (3.81, -63.5) radius 3.2512
  circle A6 centre (29.21, -63.5) radius 3.2512
  circle A7 centre (54.61, -63.5) radius 3.2512
  point P0 (0, 0)
  dimension "d41" = 6.5024
  dimension "d42" = 12.7
  dimension "d43" = 12.7
  dimension "d46" = 25.4
  constraints: 8 centre point, 1 horizontal, 14 other
  measures "d41" diameter of A0
  measures "d42" distance from line of A0.centre L0
  measures "d43" distance from line of L1 A0.centre
  measures "d46" distance of A0.centre A1.centre
extrude "Extrusion8" cut sketch "Sketch6" against normal blind 6.35
equation "\"d0\" = pd"
equation "\"d1\" = rd"
equation "\"d2\" = od"
equation "\"d3\" = a"
equation "\"d5\" = d4"
equation "\"d7\" = d6 - d4"
equation "\"d16\" = 0.5 * od"
equation "\"DP\" = 127"
equation "\"a\" = 20deg"
equation "\"ded\" = 1.25 * mod"
equation "\"od\" = pd + 2 * mod"
equation "\"rd\" = pd - 2 * ded"
equation "\"pd\" = 284.48"
equation "\"mod\" = 5.08"
body "Solid1"
